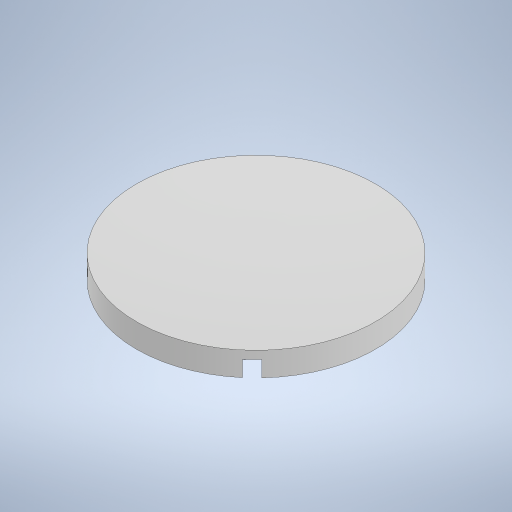
# Autodesk Inventor part: зрачок
Saved by Autodesk Inventor 2023.2 (Build 272271030, 271C)
## iProperties
Created: 2024-03-18
Part Number: зрачок
Material: Типовые
Document SubType Name: Modeling
Designer: I9232
Density: 1 g/cm^3
Appearance: По умолчанию
Author: I9232
Autodesk Inventor part; units mm, degrees
ref_plane "YZ Plane" through (0, 0, 0) normal (1, 0, 0) x (0, 1, 0)
ref_plane "XZ Plane" through (0, 0, 0) normal (0, 1, 0) x (-1, 0, 0)
ref_plane "XY Plane" through (0, 0, 0) normal (0, 0, 1) x (1, 0, 0)
sketch "Эскиз1" plane through (0, 0, 0) normal (0, 0, 1) x (1, 0, 0)
  line L0 (-15, 0) -> (-15, 3)
  line L1 (-15, 0) -> (0, 0)
  line L2 (0, 2.3791) -> (0, 0.5542) construction
  arc A0 (0, 5.3) -> (-15, 3) centre (0, -44.763) ccw
  line L3 (0, 0) -> (0, 5.3) construction
  line L4 (0, 5.3) -> (0, 0)
  dimension "d0" = 3
  dimension "d1" = 15
  dimension "d6" = 5.3
  constraints: 10 end point, 3 vertical, 2 point on circle, 1 centre point, 1 horizontal, 1 line through centre, 1 perpendicular
  measures "d0" distance of L0.start L0.end
  measures "d1" distance of L0.start L1.end
  measures "d6" distance from line of L1 L3.end
revolve "Вращение1" add sketch "Эскиз1" angle 360 about axis through (0, 5.3, 0) along (0, -1, 0)
shell "Оболочка1" thickness 0.5 removed faces 1 at (-4.7094, 0, 0) ; own thickness 0.25 on faces at (-14.9514, 2, 1.207)
fillet "Сопряжение1" radius 1 1 edges at (14.75, 2.5543, 0.0003)
sketch "Эскиз2" plane through (0, 0, 0) normal (0, -1, 0) x (1, 0, 0)
  circle A0 centre (9.875, 10.325) radius 1.1
  circle A1 centre (-9.875, 10.325) radius 1.1
  line L0 (9.875, 10.325) -> (-9.875, 10.325) construction
  line L1 (0, 10.325) -> (0, -14.875) construction
  line L2 (0, -14.875) -> (-9.875, 10.325) construction
  line L3 (0, -14.875) -> (9.875, 10.325) construction
  circle A2 centre (0, -14.875) radius 1.1
  circle A3 centre (0, 0) radius 15 projected
  line L4 (0, -15) -> (0, -14.75)
  circle A4 centre (0, 0) radius 14.75 projected
  point P0 (0, -2.275)
  point P1 (0, -2.275)
  point P2 (-9.4386, 11.3347)
  point P3 (-10.9032, 9.934)
  point P4 (10.9032, 9.934)
  point P5 (9.4386, 11.3347)
  point P6 (-10.9708, 10.2294)
  point P7 (-9.7307, 11.4155)
  point P8 (9.7307, 11.4155)
  point P9 (10.9708, 10.2294)
  point P10 (1.0875, -14.7099)
  point P11 (-1.0875, -14.7099)
  point P12 (-1.0967, -14.9599)
  point P13 (1.0967, -14.9599)
  dimension "d11" = 2.2
  dimension "d12" = 19.75
  dimension "d15" = 25.2
  constraints: 10 end point, 3 centre point, 3 coincident, 3 midpoint, 2 equal radius, 2 vertical, 1 horizontal, 4 other
  measures "d11" diameter of A0
  measures "d12" distance of L0.start L0.end
  measures "d15" vertical distance of A2.centre L0.end
extrude "Выдавливание1" cut sketch "Эскиз2" against normal blind 2 contours A0 A3 | A3 A0 A4 | A3 A1 | A1 A4 A3 | A3 L4 A4 A2 | A2 A4 L4 A3
